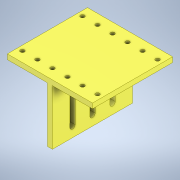
# Autodesk Inventor part: pullyBracketTopPortion
Saved by Autodesk Inventor 2022.1 (Build 261234020, 234B)
## iProperties
Created: 2021-11-10
Part Number: pullyBracketTopPortion
Material: PC/ABS Plastic
Document SubType Name: Modeling
Designer: robst
Density: 0.357273 g/cm^3
Appearance: Smooth - Yellow
Author: robst
Autodesk Inventor part; units mm, degrees
ref_plane "YZ Plane" through (0, 0, 0) normal (1, 0, 0) x (0, 1, 0)
ref_plane "XZ Plane" through (0, 0, 0) normal (0, 1, 0) x (-1, 0, 0)
ref_plane "XY Plane" through (0, 0, 0) normal (0, 0, 1) x (1, 0, 0)
sketch "Sketch1" plane through (0, 0, 0) normal (0, 1, 0) x (-1, 0, 0)
  line L0 (11.2547, 50.8) -> (-11.2547, 50.8)
  line L1 (-11.2547, 50.8) -> (-11.2547, -50.8)
  line L2 (-11.2547, -50.8) -> (11.2547, -50.8)
  line L3 (11.2547, -50.8) -> (11.2547, 50.8)
  line L4 (11.2547, 50.8) -> (-11.2547, -50.8) construction
  line L5 (-11.2547, 50.8) -> (11.2547, -50.8) construction
  point P0 (0, 0)
  dimension "d0" = 101.6
  dimension "d1" = 22.5095
  constraints: 12 end point, 2 midpoint, 2 parallel, 1 horizontal, 1 perpendicular
  measures "d0" distance of L2.end L0.start
  measures "d1" distance of L1.end L2.end
extrude "Extrusion1" add sketch "Sketch1" against normal blind 6.35
sketch "Sketch2" plane through (0, 0, 0) normal (0, 1, 0) x (1, 0, 0)
  line L0 (11.2547, -50.8) -> (-11.2547, -50.8) projected
  line L1 (-11.2547, 50.8) -> (11.2547, 50.8) projected
  line L2 (-11.2547, -50.8) -> (-4.9047, -50.8)
  line L3 (-4.9047, -50.8) -> (-4.9047, 50.8)
  line L4 (-4.9047, 50.8) -> (-11.2547, 50.8)
  line L5 (-11.2547, 50.8) -> (-11.2547, -50.8)
  point P0 (0, 0)
  dimension "d4" = 6.35
  constraints: 8 end point, 2 parallel, 1 horizontal, 1 perpendicular, 1 point on line
  measures "d4" distance between parallel lines of L3 L5
extrude "Extrusion2" add sketch "Sketch2" along normal blind 76.2
sketch "Sketch3" plane through (0, 76.2, 0) normal (0, 1, 0) x (1, 0, 0)
  line L0 (11.2547, -50.8) -> (-11.2547, -50.8) projected
  line L1 (-11.2547, -50.8) -> (-62.0547, -50.8)
  line L2 (-62.0547, -50.8) -> (-62.0547, 50.8)
  line L3 (-62.0547, 50.8) -> (-11.2547, 50.8)
  line L4 (-11.2547, 50.8) -> (-11.2547, -50.8)
  line L5 (-4.9047, -50.8) -> (-4.9047, 50.8) projected
  line L6 (-4.9047, 50.8) -> (-11.2547, 50.8) projected
  line L7 (-11.2547, -50.8) -> (-4.9047, -50.8) projected
  line L8 (11.2547, -50.8) -> (11.2547, 50.8) projected
  line L9 (11.2547, 50.8) -> (-4.9047, 50.8) projected
  line L10 (-11.2547, -50.8) -> (-11.2547, 50.8) projected
  line L11 (-11.2547, -50.8) -> (-4.9047, -50.8)
  line L12 (-4.9047, -50.8) -> (-4.9047, 50.8)
  line L13 (-4.9047, 50.8) -> (-11.2547, 50.8)
  line L14 (-11.2547, 50.8) -> (-11.2547, -50.8)
  line L15 (-4.9047, -50.8) -> (45.8953, -50.8)
  line L16 (45.8953, -50.8) -> (45.8953, 50.8)
  line L17 (45.8953, 50.8) -> (-4.9047, 50.8)
  line L18 (-4.9047, 50.8) -> (-4.9047, -50.8)
  point P0 (0, 0)
  dimension "d7" = 50.8
  dimension "d8" = 50.8
  constraints: 24 end point, 6 parallel, 3 horizontal, 3 perpendicular, 1 point on line
  measures "d7" distance of L2.end L3.end
  measures "d8" distance of L16.end L17.end
extrude "Extrusion3" add sketch "Sketch3" along normal blind 6.35
sketch "Sketch4" plane through (0, 0, 0) normal (0, 1, 0) x (1, 0, 0)
  line L0 (-4.9047, -50.8) -> (11.2547, -50.8) construction
  line L1 (3.175, -50.8) -> (3.175, 50.8) construction
  line L2 (-11.2547, 50.8) -> (11.2547, 50.8) construction
  point P0 (0, 0)
  point P1 (3.175, -38.1)
  point P2 (3.175, -12.7)
  point P3 (3.175, 12.7)
  point P4 (3.175, 38.1)
  dimension "d11" = 12.7
  dimension "d14" = 25.4
  constraints: 2 end point, 2 point on line, 2 vertical, 1 midpoint, 3 other
  measures "d11" distance from line of point (3.175, -38.1) L0
  measures "d14" distance of point (3.175, -38.1) point (3.175, -12.7)
hole "Hole1" at (3.175, 0, 38.1) at (3.175, 0, 12.7) at (3.175, 0, -12.7) at (3.175, 0, -38.1) direction (0, -1, 0) diameter 5.1054 end through all clearance for "Hex Machine Screw" size "#10" standard "Ansi Unified Screw Threads"
sketch "Sketch5" plane through (0, 82.55, 0) normal (0, 1, 0) x (1, 0, 0)
  line L0 (-62.0547, 50.8) -> (-62.0547, -50.8) construction
  line L1 (-62.0547, -38.1) -> (42.9055, -38.1) construction
  line L2 (-55.7047, -38.1) -> (-55.7047, 38.1) construction
  point P0 (0, 0)
  point P1 (-36.6547, -38.1)
  point P2 (-36.6547, 38.1)
  point P3 (-17.6047, -38.1)
  point P4 (-17.6047, 38.1)
  point P5 (1.4453, -38.1)
  point P6 (1.4453, 38.1)
  point P7 (20.4953, -38.1)
  point P8 (20.4953, 38.1)
  point P9 (39.5453, -38.1)
  point P10 (39.5453, 38.1)
  point P11 (58.5953, -38.1)
  point P12 (58.5953, 38.1)
  dimension "d26" = 38.1
  dimension "d27" = 76.2
  dimension "d28" = 6.35
  dimension "d31" = 76.2
  dimension "d34" = 19.05
  constraints: 4 end point, 2 horizontal, 2 point on line, 2 vertical, 1 coincident, 13 other
  measures "d26" distance from line of L1 point (0, 0)
  measures "d27" distance of L2.start L2.end
  measures "d28" distance between parallel lines of L2 L0
  measures "d31" distance of point (-55.705, -38.1) point (-55.705, 38.1)
  measures "d34" distance of point (-55.705, -38.1) point (-36.655, -38.1)
hole "Hole2" at (-55.7047, 82.55, 38.1) at (-55.7047, 82.55, -38.1) at (-36.6547, 82.55, 38.1) at (-36.6547, 82.55, -38.1) at (-17.6047, 82.55, 38.1) at (-17.6047, 82.55, -38.1) at (1.4453, 82.55, 38.1) at (1.4453, 82.55, -38.1) at (20.4953, 82.55, 38.1) at (20.4953, 82.55, -38.1) at (39.5453, 82.55, 38.1) at (39.5453, 82.55, -38.1) at (58.5953, 82.55, 38.1) at (58.5953, 82.55, -38.1) direction (0, -1, 0) diameter 5.1054 depth 6.35 clearance for "Hex Machine Screw" size "#10" standard "Ansi Unified Screw Threads"
sketch "Sketch8" plane through (11.2547, 0, 50.8) normal (1, 0, 0) x (0, 0, -1)
  line L0 (101.6, -6.35) -> (0, -6.35) projected
  line L1 (0, 0) -> (0, 76.2) projected
  line L2 (101.6, 0) -> (101.6, 76.2) projected
  line L3 (101.6, 0) -> (101.6, -6.35) projected
  line L4 (0, 0) -> (0, -6.35) projected
  line L5 (0, -6.35) -> (101.6, -6.35)
  line L6 (101.6, -6.35) -> (101.6, 6.35)
  line L7 (101.6, 6.35) -> (0, 6.35)
  line L8 (0, 6.35) -> (0, -6.35)
  point P0 (50.8, 0)
  point P1 (0, 6.35)
  dimension "d48" = 12.7
  constraints: 8 end point, 2 parallel, 1 horizontal, 1 perpendicular, 1 point on line
  measures "d48" distance between parallel lines of L0 L7
extrude "Extrusion5" cut sketch "Sketch8" against normal through all
sketch "Sketch9" plane through (-4.9047, 76.2, 50.8) normal (1, 0, 0) x (0, 0, -1)
  line L0 (101.6, 0) -> (0, 0) projected
  line L1 (101.6, -69.85) -> (101.6, 0) projected
  line L2 (101.6, -69.85) -> (0, -69.85) projected
  line L3 (0, -69.85) -> (0, 0) projected
  line L4 (0, -12.7) -> (101.6, -12.7) construction
  line L5 (0, -57.15) -> (101.6, -57.15) construction
  line L6 (25.4, -12.7) -> (25.4, -57.15) construction
  line L7 (22.0218, -12.7) -> (22.0218, -57.15)
  line L8 (28.7782, -57.15) -> (28.7782, -12.7)
  arc A0 (28.7782, -12.7) -> (22.0218, -12.7) centre (25.4, -12.7) ccw
  arc A1 (22.0218, -57.15) -> (28.7782, -57.15) centre (25.4, -57.15) ccw
  line L9 (50.8, -12.7) -> (50.8, -57.15) construction
  line L10 (47.4218, -12.7) -> (47.4218, -57.15)
  line L11 (54.1782, -57.15) -> (54.1782, -12.7)
  arc A2 (54.1782, -12.7) -> (47.4218, -12.7) centre (50.8, -12.7) ccw
  arc A3 (47.4218, -57.15) -> (54.1782, -57.15) centre (50.8, -57.15) ccw
  line L12 (76.2, -12.7) -> (76.2, -57.15) construction
  line L13 (72.8218, -12.7) -> (72.8218, -57.15)
  line L14 (79.5782, -57.15) -> (79.5782, -12.7)
  arc A4 (79.5782, -12.7) -> (72.8218, -12.7) centre (76.2, -12.7) ccw
  arc A5 (72.8218, -57.15) -> (79.5782, -57.15) centre (76.2, -57.15) ccw
  point P0 (50.8, -76.2)
  point P1 (25.4, -34.925)
  point P2 (50.8, -34.925)
  point P3 (76.2, -34.925)
  dimension "d51" = 12.7
  dimension "d52" = 12.7
  dimension "d53" = 25.4
  dimension "d54" = 25.4
  dimension "d55" = 25.4
  dimension "d56" = 3.3782
  constraints: 28 end point, 12 point on circle, 12 tangent, 8 point on line, 6 centre point, 6 midpoint, 5 perpendicular, 3 parallel, 2 equal radius
  measures "d51" distance from line of point (50.8, -57.15) L2
  measures "d52" distance between parallel lines of L0 L4
  measures "d53" distance between parallel lines of L6 L3
  measures "d54" distance between parallel lines of L9 L6
  measures "d55" distance between parallel lines of L12 L9
  measures "d56" radius of A0
extrude "Extrusion6" cut sketch "Sketch9" against normal through all contours A0 L8 A1 L7 | A2 L11 A3 L10 | A4 L14 A5 L13
equation "\"d0\" = BaseLength"
equation "\"d1\" = BaseWidth"
equation "\"d2\" = BaseThickness"
equation "\"d4\" = BackWidth"
equation "\"d5\" = BackHeight"
equation "\"d7\" = TopBackExtension"
equation "\"d8\" = TopFrontExtension"
equation "\"d9\" = TopThickness"
equation "\"d11\" = offsetForFirstHole"
equation "\"d26\" = 0.5 * holeSpacingForMotorBracket"
equation "\"d27\" = holeSpacingForMotorBracket"
equation "\"d28\" = offsetForBracketHoleFromEdge"
equation "\"d34\" = holeSpacingForVariationInMotorBracketHoles"
equation "\"BaseWidth\" = 22.50948"
equation "\"BaseLength\" = 101.6"
equation "\"BaseThickness\" = 6.35"
equation "\"BackWidth\" = 6.35"
equation "\"BackHeight\" = 76.2"
equation "\"TopBackExtension\" = 50.8"
equation "\"TopFrontExtension\" = 50.8"
equation "\"TopThickness\" = 6.35"
equation "\"offsetForFirstHole\" = 12.7"
equation "\"holeSpacingForMotorBracket\" = 76.2"
equation "\"offsetForBracketHoleFromEdge\" = 6.35"
equation "\"holeSpacingForVariationInMotorBracketHoles\" = 19.05"
equation "\"deltaForSlots\" = 0.25 * BaseLength"
body "Solid1"
